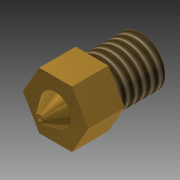
# Autodesk Inventor part: ChimeraNozzle.4
Saved by Autodesk Inventor 2015 (Build 190159000, 159)
## iProperties
Created: 2014-08-17
Part Number: ChimeraNozzle.4
Material: Brass, Soft Yellow
Document SubType Name: Modeling
Designer: Jack
Density: 8.47 g/cm^3
Appearance: Brass - Satin
Author: Jack
Autodesk Inventor part; units mm, degrees
ref_plane "YZ Plane" through (0, 0, 0) normal (1, 0, 0) x (0, 1, 0)
ref_plane "XZ Plane" through (0, 0, 0) normal (0, 1, 0) x (-1, 0, 0)
ref_plane "XY Plane" through (0, 0, 0) normal (0, 0, 1) x (1, 0, 0)
sketch "Sketch1" plane through (0, 0, 0) normal (0, 0, 1) x (1, 0, 0)
  line L0 (0, 0) -> (0.5, 0)
  line L1 (0.5, 0) -> (1.9004, 2)
  line L2 (1.9004, 2) -> (4.5, 2)
  line L3 (4.5, 2) -> (4.5, 5)
  line L4 (4.5, 5) -> (2.5, 5)
  line L5 (2.5, 5) -> (2.5, 6.5)
  line L6 (2.5, 6.5) -> (3, 6.5)
  line L7 (3, 6.5) -> (3, 12.5)
  line L8 (3, 12.5) -> (0, 12.5)
  line L9 (0, 12.5) -> (0, 0)
  dimension "d0" = 0.5
  dimension "d1" = 125
  dimension "d3" = 4.5
  dimension "d4" = 3
  dimension "d5" = 2.5
  dimension "d6" = 1.5
  dimension "d7" = 3
  dimension "d8" = 10.5
  dimension "d9" = 12.5
  constraints: 20 end point, 4 perpendicular, 3 vertical, 2 horizontal
  measures "d0" distance of L0.start L0.end
  measures "d1" angle of L0 L1
  measures "d3" horizontal distance of L0.start L2.end
  measures "d4" distance of L2.end L3.end
  measures "d5" horizontal distance of L0.start L4.end
  measures "d6" distance of L4.end L5.end
  measures "d7" horizontal distance of L0.start L6.end
  measures "d8" distance between parallel lines of L2 L8
  measures "d9" distance between parallel lines of L0 L8
revolve "Revolution1" add sketch "Sketch1" angle 360 about axis through (0, 12.5, 0) along (0, -1, 0)
sketch "Sketch2" plane through (0, 5, 0) normal (0, 1, 0) x (1, 0, 0)
  circle A0 centre (0, 0) radius 4.5 projected
  line L0 (4.0415, 0) -> (2.0207, -3.5)
  line L1 (2.0207, -3.5) -> (-2.0207, -3.5)
  line L2 (-2.0207, -3.5) -> (-4.0415, 0)
  line L3 (-4.0415, 0) -> (-2.0207, 3.5)
  line L4 (-2.0207, 3.5) -> (2.0207, 3.5)
  line L5 (2.0207, 3.5) -> (4.0415, 0)
  dimension "d11" = 7
  constraints: 12 end point, 1 coincident, 1 horizontal, 13 other
  measures "d11" distance between parallel lines of L4 L1
extrude "Extrusion1" cut sketch "Sketch2" against normal up to surface (3 mm away)
thread "Thread1" size "M6x1" class "6g" standard "ANSI Metric M Profile" full length
sketch "Sketch3" plane through (0, 12.5, 0) normal (0, 1, 0) x (1, 0, 0)
  circle A0 centre (0, 0) radius 3 projected
  circle A1 centre (0, 0) radius 1
  dimension "d16" = 2
  constraints: 1 centre point, 1 coincident
  measures "d16" diameter of A1
extrude "Extrusion2" cut sketch "Sketch3" against normal blind 10.5 contours A1
sketch "Sketch4" plane through (0, 0, 0) normal (0, -1, 0) x (1, 0, 0)
  circle A0 centre (0, 0) radius 0.5 projected
  circle A1 centre (0, 0) radius 0.2
  dimension "d19" = 0.4
  constraints: 1 centre point, 1 coincident
  measures "d19" diameter of A1
extrude "Extrusion3" cut sketch "Sketch4" against normal up to surface (2 mm away) contours A1
body "Solid1"
